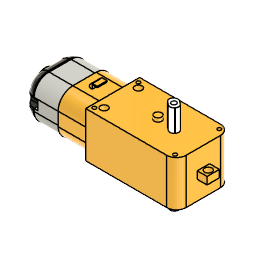
DC Motor (Autodesk Fusion 360 design; units mm, degrees)
part number: 2025-10-12-13-39-24-914
part number: 2025-10-12-13-42-40-722
part number: 2025-10-12-13-44-59-312
part number: 2025-10-12-15-17-17-342
part number: 2025-10-12-15-31-43-485
part number: 2025-10-12-15-34-23-255
part number: 2025-10-12-15-55-27-958
part number: 2025-10-12-16-01-49-874
Autodesk Fusion 360 part; units mm, degrees
sketch "Sketch1" plane through (0, 0, 0) normal (0, 1, 0) x (1, 0, 0)
  line L0 (18.5, 9.25) -> (-18.5, 9.25)
  line L1 (-18.5, 9.25) -> (-18.5, -9.25)
  line L2 (-18.5, -9.25) -> (18.5, -9.25)
  line L3 (18.5, -9.25) -> (18.5, 9.25)
  line L4 (18.5, 9.25) -> (-18.5, -9.25) construction
  line L5 (-18.5, 9.25) -> (18.5, -9.25) construction
  dimension "d1" = 37
  dimension "d2" = 18.5
  constraint horizontal L0
  constraint perpendicular L0 L1
  constraint parallel L0 L2
  constraint parallel L1 L3
  constraint coincident L4 origin
  constraint coincident L5 origin
  measures "d1" distance of L1.end L2.end
  measures "d2" distance of L0.start L2.end
extrude "Extrude1" add sketch "Sketch1" along normal blind 22 makes body 1
sketch "Sketch2" plane through (-18.5, 0, 0) normal (-1, 0, 0) x (0, -1, 0)
  line L0 (0, -9.25) -> (0, 9.25)
  line L1 (0, 9.25) -> (-22, 9.25)
  line L2 (-22, 9.25) -> (-22, -9.25)
  line L3 (-22, -9.25) -> (0, -9.25)
  line L4 (-0.25, -9.05) -> (-21.75, -9.05)
  line L5 (-21.75, -9.05) -> (-21.75, 8.45)
  line L6 (-21.75, 8.45) -> (-0.25, 8.45)
  line L7 (-0.25, 8.45) -> (-0.25, -9.05)
  line L8 (-0.25, -9.05) -> (-21.75, 8.45) construction
  line L9 (-21.75, -9.05) -> (-0.25, 8.45) construction
  point P0 (-11, -0.3)
  dimension "d5" = 21.5
  dimension "d6" = 17.5
  dimension "d7" = 0.25
  dimension "d8" = 0.2
  constraint horizontal L4
  constraint perpendicular L4 L5
  constraint parallel L4 L6
  constraint parallel L5 L7
  constraint coincident L8 P0
  constraint coincident L9 P0
  measures "d5" distance of L5.end L6.end
  measures "d6" distance of L4.start L6.end
  measures "d7" distance of L2 L5
  measures "d8" distance of L3 L4
extrude "Extrude1'" add sketch "Sketch2" along normal blind 11.5 separate body contours L4 L5 L6 L7 makes body 2 in component "Component"
sketch "Sketch3" plane through (-30, 0, 0) normal (-1, 0, 0) x (0, -1, 0)
  line L0 (-0.25, 8.45) -> (-21.75, 8.45)
  line L1 (-21.75, 8.45) -> (-21.75, -9.05)
  line L2 (-21.75, -9.05) -> (-0.25, -9.05)
  line L3 (-0.25, -9.05) -> (-0.25, 8.45)
  line L4 (-0.454, -8.785) -> (-21.454, -8.785)
  line L5 (-21.454, -8.785) -> (-21.454, 8.215)
  line L6 (-21.454, 8.215) -> (-0.454, 8.215)
  line L7 (-0.454, 8.215) -> (-0.454, -8.785)
  line L8 (-0.454, -8.785) -> (-21.454, 8.215) construction
  line L9 (-21.454, -8.785) -> (-0.454, 8.215) construction
  point P0 (-10.954, -0.285)
  dimension "d11" = 21
  dimension "d12" = 17
  dimension "d13" = 0.235
  dimension "d14" = 0.296
  constraint horizontal L4
  constraint perpendicular L4 L5
  constraint parallel L4 L6
  constraint parallel L5 L7
  constraint coincident L8 P0
  constraint coincident L9 P0
  measures "d11" distance of L5.end L6.end
  measures "d12" distance of L4.start L6.end
  measures "d13" distance of L0 L6
  measures "d14" distance of L1 L5
extrude "Extrude1''" add sketch "Sketch3" along normal blind 10 separate body contours L4 L5 L6 L7 makes body 3 in component "Component'"
fillet "Fillet1" radius 4 2 edges at (18.5, 0, 0) (18.5, 22, 0) on bodies 1
sketch "Sketch4" plane through (18.5, 0, 0) normal (1, 0, 0) x (0, 1, 0)
  line L0 (18, -9.25) -> (18, 9.25)
  line L1 (18, 9.25) -> (4, 9.25)
  line L2 (4, 9.25) -> (4, -9.25)
  line L3 (4, -9.25) -> (18, -9.25)
  line L4 (13.5, -1.5) -> (8.5, -1.5)
  line L5 (8.5, -1.5) -> (8.5, 1.5)
  line L6 (8.5, 1.5) -> (13.5, 1.5)
  line L7 (13.5, 1.5) -> (13.5, -1.5)
  line L8 (13.5, -1.5) -> (8.5, 1.5) construction
  line L9 (8.5, -1.5) -> (13.5, 1.5) construction
  point P0 (11, 0)
  dimension "d23" = 5
  dimension "d24" = 3
  constraint horizontal L4
  constraint perpendicular L4 L5
  constraint parallel L4 L6
  constraint parallel L5 L7
  constraint coincident L8 P0
  constraint coincident L9 P0
  measures "d23" distance of L5.end L6.end
  measures "d24" distance of L4.start L6.end
extrude "Extrude2" add sketch "Sketch4" along normal blind 4 contours L4 L5 L6 L7 bodies 1
sketch "Sketch5" plane through (0, 0, 1.5) normal (0, 0, 1) x (-1, 0, 0)
  line L0 (-18.5, -13.5) -> (-18.5, -8.5)
  line L1 (-18.5, -8.5) -> (-22.5, -8.5)
  line L2 (-22.5, -8.5) -> (-22.5, -13.5)
  line L3 (-22.5, -13.5) -> (-18.5, -13.5)
  circle A0 centre (-20.5, -11) radius 1.5
  dimension "d27" = 3
  measures "d27" diameter of A0
extrude "Extrude3" cut sketch "Sketch5" against normal blind 3 contours A0 bodies 1
sketch "Sketch7" plane through (0, 0, 9.25) normal (0, 0, 1) x (-1, 0, 0)
  arc A0 (-18.5, -18) -> (-14.5, -22) centre (-14.5, -18) ccw
  line L0 (-14.5, -22) -> (18.5, -22)
  line L1 (18.5, -22) -> (18.5, 0)
  line L2 (18.5, 0) -> (-14.5, 0)
  arc A1 (-14.5, 0) -> (-18.5, -4) centre (-14.5, -4) ccw
  line L3 (-18.5, -4) -> (-18.5, -18)
  line L4 (-7.3842, -8.0793) -> (-3.453, -11.169)
  line L5 (-3.453, -11.169) -> (-5.6158, -13.9207)
  line L6 (-5.6158, -13.9207) -> (-9.547, -10.831)
  line L7 (-9.547, -10.831) -> (-7.3842, -8.0793)
  line L8 (-7.3842, -8.0793) -> (-5.6158, -13.9207) construction
  line L9 (-3.453, -11.169) -> (-9.547, -10.831) construction
  point P0 (-6.5, -11)
  dimension "d32" = 5
  dimension "d33" = 3.5
  dimension "d34" = 12
  dimension "d35" = 11
  constraint perpendicular L4 L5
  constraint parallel L4 L6
  constraint parallel L5 L7
  constraint coincident L8 P0
  constraint coincident L9 P0
  measures "d32" distance of L5.end L6.end
  measures "d33" distance of L4.start L6.end
  measures "d34" distance of L3 P0
  measures "d35" distance of L2 P0
extrude "Extrude4" add sketch "Sketch7" along normal blind 9 separate body contours L4 L5 L6 L7 makes body 4
extrude "Extrude5" add 1 faces at (5.4843, 11.0563, 18.25) along direction (0, 0, -1) blind 36.5 on bodies 4 bodies 1 4
fillet "Fillet2" radius 1.65 8 edges at (7.3842, 8.0793, 13.75) (9.547, 10.831, 13.75) (3.453, 11.169, 13.75) (5.6158, 13.9207, 13.75) (9.547, 10.831, -13.75) (5.6158, 13.9207, -13.75) (3.453, 11.169, -13.75) (7.3842, 8.0793, -13.75) on bodies 1
sketch "Sketch8" plane through (0, 0, 9.25) normal (0, 0, 1) x (-1, 0, 0)
  line L0 (-8.5274, -9.5338) -> (-8.4038, -9.3765)
  arc A0 (-6.0869, -9.0989) -> (-8.4038, -9.3765) centre (-7.1065, -10.3961) ccw
  line L1 (-6.0869, -9.0989) -> (-4.7503, -10.1494)
  arc A1 (-4.4726, -12.4662) -> (-4.7503, -10.1494) centre (-5.7699, -11.4466) ccw
  line L2 (-4.4726, -12.4662) -> (-4.5962, -12.6235)
  arc A2 (-6.9131, -12.9011) -> (-4.5962, -12.6235) centre (-5.8935, -11.6039) ccw
  line L3 (-6.9131, -12.9011) -> (-8.2497, -11.8506)
  arc A3 (-8.5274, -9.5338) -> (-8.2497, -11.8506) centre (-7.2301, -10.5534) ccw
  arc A4 (-18.5, -18) -> (-14.5, -22) centre (-14.5, -18) ccw
  line L4 (-14.5, -22) -> (18.5, -22)
  line L5 (18.5, -22) -> (18.5, 0)
  line L6 (18.5, 0) -> (-14.5, 0)
  arc A5 (-14.5, 0) -> (-18.5, -4) centre (-14.5, -4) ccw
  line L7 (-18.5, -4) -> (-18.5, -18)
  circle A6 centre (17, -20) radius 0.75
  circle A7 centre (-16, -20) radius 0.75
  circle A8 centre (-16, -2) radius 0.75
  circle A9 centre (17, -2) radius 0.75
  dimension "d42" = 1.5
  dimension "d43" = 1.5
  dimension "d44" = 1.5
  dimension "d45" = 1.5
  measures "d42" diameter of A6
  measures "d43" diameter of A7
  measures "d44" diameter of A8
  measures "d45" diameter of A9
extrude "Extrude6" cut sketch "Sketch8" against normal blind 5 contours A6 | A7 | A8 | A9 bodies 1
sketch "Sketch9" plane through (0, 0, 9.25) normal (0, 0, 1) x (-1, 0, 0)
  circle A0 centre (-16, -20) radius 0.75
  circle A1 centre (-16, -2) radius 0.75
  circle A2 centre (17, -20) radius 0.75
  circle A3 centre (17, -2) radius 0.75
  line L0 (-8.5274, -9.5338) -> (-8.4038, -9.3765)
  arc A4 (-6.0869, -9.0989) -> (-8.4038, -9.3765) centre (-7.1065, -10.3961) ccw
  line L1 (-6.0869, -9.0989) -> (-4.7503, -10.1494)
  arc A5 (-4.4726, -12.4662) -> (-4.7503, -10.1494) centre (-5.7699, -11.4466) ccw
  line L2 (-4.4726, -12.4662) -> (-4.5962, -12.6235)
  arc A6 (-6.9131, -12.9011) -> (-4.5962, -12.6235) centre (-5.8935, -11.6039) ccw
  line L3 (-6.9131, -12.9011) -> (-8.2497, -11.8506)
  arc A7 (-8.5274, -9.5338) -> (-8.2497, -11.8506) centre (-7.2301, -10.5534) ccw
  arc A8 (-18.5, -18) -> (-14.5, -22) centre (-14.5, -18) ccw
  line L4 (-14.5, -22) -> (18.5, -22)
  line L5 (18.5, -22) -> (18.5, 0)
  line L6 (18.5, 0) -> (-14.5, 0)
  arc A9 (-14.5, 0) -> (-18.5, -4) centre (-14.5, -4) ccw
  line L7 (-18.5, -4) -> (-18.5, -18)
  circle A10 centre (15, -18) radius 1.5
  circle A11 centre (-14, -18) radius 1.5
  circle A12 centre (-14, -4) radius 1.5
  circle A13 centre (15, -4) radius 1.5
  dimension "d48" = 3
  dimension "d49" = 3
  dimension "d50" = 3
  dimension "d51" = 3
  measures "d48" diameter of A10
  measures "d49" diameter of A11
  measures "d50" diameter of A12
  measures "d51" diameter of A13
extrude "Extrude7" cut sketch "Sketch9" against normal blind 5 contours A10 | A13 bodies 1
extrude "Extrude8" cut 2 faces at (-15.3832, 18.562, 4.25) (-15.237, 3.6091, 4.25) along direction (0, 0, -1) blind 10 on bodies 1 bodies 1
extrude "Extrude9" cut 2 faces at (-15.3832, 18.562, -5.75) (-15.237, 3.6091, -5.75) along direction (0, 0, -1) blind 25 on bodies 1 bodies 1
sketch "Sketch10" plane through (0, 0, -9.25) normal (0, 0, -1) x (1, 0, 0)
  circle A0 centre (-15, -18) radius 1.5
  circle A1 centre (-15, -4) radius 1.5
  line L0 (4.5962, -12.6235) -> (4.4726, -12.4662)
  arc A2 (4.7503, -10.1494) -> (4.4726, -12.4662) centre (5.7699, -11.4466) ccw
  line L1 (4.7503, -10.1494) -> (6.0869, -9.0989)
  arc A3 (8.4038, -9.3765) -> (6.0869, -9.0989) centre (7.1065, -10.3961) ccw
  line L2 (8.4038, -9.3765) -> (8.5274, -9.5338)
  arc A4 (8.2497, -11.8506) -> (8.5274, -9.5338) centre (7.2301, -10.5534) ccw
  line L3 (8.2497, -11.8506) -> (6.9131, -12.9011)
  arc A5 (4.5962, -12.6235) -> (6.9131, -12.9011) centre (5.8935, -11.6039) ccw
  arc A6 (14.5, -22) -> (18.5, -18) centre (14.5, -18) ccw
  line L4 (18.5, -18) -> (18.5, -4)
  arc A7 (18.5, -4) -> (14.5, 0) centre (14.5, -4) ccw
  line L5 (14.5, 0) -> (-18.5, 0)
  line L6 (-18.5, 0) -> (-18.5, -22)
  line L7 (-18.5, -22) -> (14.5, -22)
  circle A8 centre (-16.4, -6.9) radius 2
  circle A9 centre (-16.4, -15.1) radius 2
  dimension "d58" = 4
  dimension "d59" = 4
  measures "d58" diameter of A8
  measures "d59" diameter of A9
extrude "Extrude10" cut sketch "Sketch10" against normal blind 3 contours A0 A9 | A1 A8 picked at (-16.6375, -14.3779) picked at (-16.6375, -7.6221) bodies 1
sketch "Sketch11" plane through (-40, 0, 0) normal (-1, 0, 0) x (0, -1, 0)
  line L0 (-0.454, 8.215) -> (-21.454, 8.215)
  line L1 (-21.454, 8.215) -> (-21.454, -8.785)
  line L2 (-21.454, -8.785) -> (-0.454, -8.785)
  line L3 (-0.454, -8.785) -> (-0.454, 8.215)
  line L4 (-0.654, -8.685) -> (-21.254, -8.685)
  line L5 (-21.254, -8.685) -> (-21.254, 8.115)
  line L6 (-21.254, 8.115) -> (-0.654, 8.115)
  line L7 (-0.654, 8.115) -> (-0.654, -8.685)
  line L8 (-0.654, -8.685) -> (-21.254, 8.115) construction
  line L9 (-21.254, -8.685) -> (-0.654, 8.115) construction
  point P0 (-10.954, -0.285)
  dimension "d62" = 0.1
  dimension "d63" = 0.2
  dimension "d64" = 0.2
  dimension "d65" = 0.1
  constraint horizontal L4
  constraint perpendicular L4 L5
  constraint parallel L4 L6
  constraint parallel L5 L7
  constraint coincident L8 P0
  constraint coincident L9 P0
  measures "d62" distance of L0 L6
  measures "d63" distance of L3 L7
  measures "d64" distance of L1 L5
  measures "d65" distance of L2 L4
extrude "Extrude1'''" add sketch "Sketch11" along normal blind 4 separate body contours L4 L5 L6 L7 makes body 5 in component "Component''"
sketch "Sketch12" plane through (0, 21.454, 0) normal (0, 1, 0) x (-1, 0, 0)
  line L0 (30, 8.215) -> (30, -8.785)
  line L1 (30, -8.785) -> (40, -8.785)
  line L2 (40, -8.785) -> (40, 8.215)
  line L3 (40, 8.215) -> (30, 8.215)
  line L4 (45.5, -1.75) -> (38.5, -1.75)
  line L5 (38.5, -1.75) -> (38.5, 1.75)
  line L6 (38.5, 1.75) -> (45.5, 1.75)
  line L7 (45.5, 1.75) -> (45.5, -1.75)
  line L8 (45.5, -1.75) -> (38.5, 1.75) construction
  line L9 (38.5, -1.75) -> (45.5, 1.75) construction
  point P0 (42, 0)
  dimension "d68" = 7
  dimension "d69" = 3.5
  constraint horizontal L4
  constraint perpendicular L4 L5
  constraint parallel L4 L6
  constraint parallel L5 L7
  constraint coincident L8 P0
  constraint coincident L9 P0
  measures "d68" distance of L5.end L6.end
  measures "d69" distance of L4.start L6.end
extrude "Extrude2'" cut sketch "Sketch12" against normal blind 2.5 contours L2 L4 L6 L7 | L2 L4 L5 L6 bodies 3 in component "Component'"
extrude "Extrude2''" cut sketch "Sketch12" against normal blind 2.5 contours L2 L4 L6 L7 | L2 L4 L5 L6 bodies 5 in component "Component''"
sketch "Sketch13" plane through (0, 0.454, 0) normal (0, -1, 0) x (1, 0, 0)
  line L0 (-30, -8.785) -> (-30, 8.215)
  line L1 (-30, 8.215) -> (-40, 8.215)
  line L2 (-40, 8.215) -> (-40, -8.785)
  line L3 (-40, -8.785) -> (-30, -8.785)
  line L4 (-38.4787, -1.7463) -> (-45.4787, -1.7463)
  line L5 (-45.4787, -1.7463) -> (-45.4787, 1.7537)
  line L6 (-45.4787, 1.7537) -> (-38.4787, 1.7537)
  line L7 (-38.4787, 1.7537) -> (-38.4787, -1.7463)
  line L8 (-38.4787, -1.7463) -> (-45.4787, 1.7537) construction
  line L9 (-45.4787, -1.7463) -> (-38.4787, 1.7537) construction
  point P0 (-41.9787, 0.0037)
  dimension "d74" = 7
  dimension "d75" = 3.5
  constraint horizontal L4
  constraint perpendicular L4 L5
  constraint parallel L4 L6
  constraint parallel L5 L7
  constraint coincident L8 P0
  constraint coincident L9 P0
  measures "d74" distance of L5.end L6.end
  measures "d75" distance of L4.start L6.end
extrude "Extrude3'" cut sketch "Sketch13" against normal blind 2.5 contours L2 L4 L5 L6 | L2 L4 L6 L7 bodies 3 in component "Component'"
extrude "Extrude3''" cut sketch "Sketch13" against normal blind 2.5 contours L2 L4 L5 L6 | L2 L4 L6 L7 bodies 5 in component "Component''"
fillet "Fillet2'" radius 6 4 edges at (-35, 0.454, 8.215) (-35, 21.454, 8.215) (-35, 21.454, -8.785) (-35, 0.454, -8.785) on bodies 3 in component "Component'"
fillet "Fillet1'" radius 6 4 edges at (-42, 0.654, 8.115) (-42, 0.654, -8.685) (-42, 21.254, 8.115) (-42, 21.254, -8.685) on bodies 5 in component "Component''"
fillet "Fillet2''" radius 6 4 edges at (-24.25, 0.25, 8.45) (-24.25, 0.25, -9.05) (-24.25, 21.75, 8.45) (-24.25, 21.75, -9.05) on bodies 2 in component "Component"
sketch "Sketch14" plane through (-44, 0, 0) normal (-1, 0, 0) x (0, -1, 0)
  arc A0 (-21.254, -2.685) -> (-15.254, -8.685) centre (-15.254, -2.685) ccw
  line L0 (-15.254, -8.685) -> (-6.654, -8.685)
  arc A1 (-6.654, -8.685) -> (-0.654, -2.685) centre (-6.654, -2.685) ccw
  line L1 (-0.654, -2.685) -> (-0.654, -1.7463)
  line L2 (-0.654, -1.7463) -> (-2.954, -1.7463)
  line L3 (-2.954, -1.7463) -> (-2.954, 1.7537)
  line L4 (-2.954, 1.7537) -> (-0.654, 1.7537)
  line L5 (-0.654, 1.7537) -> (-0.654, 2.115)
  arc A2 (-0.654, 2.115) -> (-6.654, 8.115) centre (-6.654, 2.115) ccw
  line L6 (-6.654, 8.115) -> (-15.254, 8.115)
  arc A3 (-15.254, 8.115) -> (-21.254, 2.115) centre (-15.254, 2.115) ccw
  line L7 (-21.254, 2.115) -> (-21.254, 1.75)
  line L8 (-21.254, 1.75) -> (-18.954, 1.75)
  line L9 (-18.954, 1.75) -> (-18.954, -1.75)
  line L10 (-18.954, -1.75) -> (-21.254, -1.75)
  line L11 (-21.254, -1.75) -> (-21.254, -2.685)
  circle A4 centre (-11, 0) radius 4.5
  dimension "d86" = 9
  measures "d86" diameter of A4
extrude "Extrude1''''" add sketch "Sketch14" along normal blind 2 separate body contours A4 makes body 6 in component "Component'''"
sketch "Sketch15" plane through (-46, 0, 0) normal (-1, 0, 0) x (0, -1, 0)
  circle A0 centre (-11, 0) radius 4.5
  circle A1 centre (-11, 0) radius 1.5
  dimension "d89" = 3
  constraint concentric A0 A1
  measures "d89" diameter of A1
extrude "Extrude2'''" cut sketch "Sketch15" against normal blind 1 contours A1 bodies 6 in component "Component'''"
sketch "Sketch16" plane through (-45, 0, 0) normal (-1, 0, 0) x (0, -1, 0)
  circle A0 centre (-11, 0) radius 1.5
  circle A1 centre (-11, 0) radius 0.5
  dimension "d92" = 1
  constraint concentric A0 A1
  measures "d92" diameter of A1
extrude "Extrude1'''''" add sketch "Sketch16" along normal blind 2 separate body contours A1 makes body 7 in component "Component''''"
sketch "Sketch17" plane through (-46, 0, 0) normal (-1, 0, 0) x (0, -1, 0)
  circle A0 centre (-11, 0) radius 1.5
  circle A1 centre (-11, 0) radius 4.5
  line L0 (-8.2595, 2.0042) -> (-13.7595, 2.0042)
  line L1 (-13.7595, 2.0042) -> (-13.7595, 3.0042)
  line L2 (-13.7595, 3.0042) -> (-8.2595, 3.0042)
  line L3 (-8.2595, 3.0042) -> (-8.2595, 2.0042)
  line L4 (-8.2595, 2.0042) -> (-13.7595, 3.0042) construction
  line L5 (-13.7595, 2.0042) -> (-8.2595, 3.0042) construction
  point P0 (-11.0095, 2.5042)
  dimension "d95" = 5.5
  dimension "d96" = 1
  constraint horizontal L0
  constraint perpendicular L0 L1
  constraint parallel L0 L2
  constraint parallel L1 L3
  constraint coincident L4 P0
  constraint coincident L5 P0
  measures "d95" distance of L1.end L2.end
  measures "d96" distance of L0.end L1.end
extrude "Extrude4'" cut sketch "Sketch17" against normal blind 3 contours L0 L1 L2 L3 bodies 5 in component "Component''"
extrude "Extrude3'''" cut sketch "Sketch17" against normal blind 3 contours L0 L1 L2 L3 bodies 6 in component "Component'''"
sketch "Sketch18" plane through (-46, 0, 0) normal (-1, 0, 0) x (0, -1, 0)
  line L0 (-13.7595, 2.0042) -> (-13.7595, 3.0042)
  line L1 (-13.7595, 3.0042) -> (-8.2595, 3.0042)
  line L2 (-8.2595, 3.0042) -> (-8.2595, 2.0042)
  line L3 (-8.2595, 2.0042) -> (-13.7595, 2.0042)
  circle A0 centre (-11, 0) radius 1.5
  circle A1 centre (-11, 0) radius 4.5
  line L4 (-14.0414, -3.3166) -> (-7.9586, -3.3166)
  constraint coincident A1 L4.start
  constraint coincident A1 L4.end
  constraint horizontal L4
extrude "Extrude4''" cut sketch "Sketch18" against normal blind 2 contours A1 L4 picked at (-11.8392, -3.4544) bodies 6 in component "Component'''"
fillet "Fillet2'''" radius 3.5 10 edges at (-44, 21.254, 1.9325) (-44, 19.4966, 6.3576) (-44, 10.954, 8.115) (-44, 2.4114, 6.3576) (-44, 0.654, 1.9344) (-44, 0.654, -2.2156) (-44, 2.4114, -6.9276) (-44, 10.954, -8.685) (-44, 19.4966, -6.9276) (-44, 21.254, -2.2175) on bodies 5 in component "Component''"
sketch "Sketch19" plane through (0, 0, 8.45) normal (0, 0, 1) x (-1, 0, 0)
  line L0 (18.5, -15.75) -> (30, -15.75)
  line L1 (30, -15.75) -> (30, -6.25)
  line L2 (30, -6.25) -> (18.5, -6.25)
  line L3 (18.5, -6.25) -> (18.5, -15.75)
  line L4 (26, -13.0103) -> (24.8, -13.0103)
  line L5 (24.8, -13.0103) -> (24.8, -9.0103)
  line L6 (24.8, -9.0103) -> (26, -9.0103)
  line L7 (26, -9.0103) -> (26, -13.0103)
  line L8 (26, -13.0103) -> (24.8, -9.0103) construction
  line L9 (24.8, -13.0103) -> (26, -9.0103) construction
  point P0 (25.4, -11.0103)
  dimension "d105" = 4
  dimension "d106" = 4
  dimension "d107" = 1.2
  constraint horizontal L4
  constraint perpendicular L4 L5
  constraint parallel L4 L6
  constraint parallel L5 L7
  constraint coincident L8 P0
  constraint coincident L9 P0
  measures "d105" distance of L4.end L5.end
  measures "d106" distance of L1 L7
  measures "d107" distance of L5.end L6.end
extrude "Extrude2''''" add sketch "Sketch19" along normal blind 2 contours L4 L5 L6 L7 bodies 2 in component "Component"
sketch "Sketch20" plane through (-24.8, 0, 0) normal (1, 0, 0) x (0, 1, 0)
  line L0 (9.0103, 8.45) -> (13.0103, 8.45)
  line L1 (13.0103, 8.45) -> (13.0103, 10.45)
  line L2 (13.0103, 10.45) -> (9.0103, 10.45)
  line L3 (9.0103, 10.45) -> (9.0103, 8.45)
  line L4 (13.0147, 9.949) -> (9.0147, 9.949)
  line L5 (9.0147, 9.949) -> (9.0147, 10.449)
  line L6 (9.0147, 10.449) -> (13.0147, 10.449)
  line L7 (13.0147, 10.449) -> (13.0147, 9.949)
  line L8 (13.0147, 9.949) -> (9.0147, 10.449) construction
  line L9 (9.0147, 9.949) -> (13.0147, 10.449) construction
  point P0 (11.0147, 10.199)
  dimension "d110" = 4
  dimension "d111" = 0.5
  dimension "d112" = 0.001
  constraint horizontal L4
  constraint perpendicular L4 L5
  constraint parallel L4 L6
  constraint parallel L5 L7
  constraint coincident L8 P0
  constraint coincident L9 P0
  measures "d110" distance of L5.end L6.end
  measures "d111" distance of L4.end L5.end
  measures "d112" distance of L2 L6
extrude "Extrude3''''" add sketch "Sketch20" along normal blind 2 contours L1 L4 L5 L6 bodies 2 in component "Component"
chamfer "Chamfer1" distance 1 angle 45 1 edges at (-26, 11.0103, 10.45) on bodies 2 in component "Component"
sketch "Sketch21" plane through (0, 0, -9.05) normal (0, 0, -1) x (1, 0, 0)
  line L0 (-30, -15.75) -> (-18.5, -15.75)
  line L1 (-18.5, -15.75) -> (-18.5, -6.25)
  line L2 (-18.5, -6.25) -> (-30, -6.25)
  line L3 (-30, -6.25) -> (-30, -15.75)
  line L4 (-26, -9.0505) -> (-24.8, -9.0505)
  line L5 (-24.8, -9.0505) -> (-24.8, -13.0505)
  line L6 (-24.8, -13.0505) -> (-26, -13.0505)
  line L7 (-26, -13.0505) -> (-26, -9.0505)
  line L8 (-26, -9.0505) -> (-24.8, -13.0505) construction
  line L9 (-24.8, -9.0505) -> (-26, -13.0505) construction
  point P0 (-25.4, -11.0505)
  dimension "d116" = 4
  dimension "d117" = 1.2
  dimension "d118" = 4
  constraint horizontal L4
  constraint perpendicular L4 L5
  constraint parallel L4 L6
  constraint parallel L5 L7
  constraint coincident L8 P0
  constraint coincident L9 P0
  measures "d116" distance of L4.start L6.end
  measures "d117" distance of L4.start L4.end
  measures "d118" distance of L3 L7
extrude "Extrude4'''" add sketch "Sketch21" along normal blind 2 contours L4 L5 L6 L7 bodies 2 in component "Component"
sketch "Sketch22" plane through (-24.8, 0, 0) normal (1, 0, 0) x (0, 1, 0)
  line L0 (13.0505, -9.05) -> (9.0505, -9.05)
  line L1 (9.0505, -9.05) -> (9.0505, -11.05)
  line L2 (9.0505, -11.05) -> (13.0505, -11.05)
  line L3 (13.0505, -11.05) -> (13.0505, -9.05)
  line L4 (9.0605, -10.544) -> (13.0605, -10.544)
  line L5 (13.0605, -10.544) -> (13.0605, -11.044)
  line L6 (13.0605, -11.044) -> (9.0605, -11.044)
  line L7 (9.0605, -11.044) -> (9.0605, -10.544)
  line L8 (9.0605, -10.544) -> (13.0605, -11.044) construction
  line L9 (13.0605, -10.544) -> (9.0605, -11.044) construction
  point P0 (11.0605, -10.794)
  dimension "d121" = 4
  dimension "d122" = 0.5
  constraint horizontal L4
  constraint perpendicular L4 L5
  constraint parallel L4 L6
  constraint parallel L5 L7
  constraint coincident L8 P0
  constraint coincident L9 P0
  measures "d121" distance of L5.end L6.end
  measures "d122" distance of L4.start L6.end
extrude "Extrude5'" add sketch "Sketch22" along normal blind 2 contours L3 L4 L6 L7 bodies 2 in component "Component"
chamfer "Chamfer2" distance 1 angle 45 1 edges at (-26, 11.0505, -11.05) on bodies 2 in component "Component"
sketch "Sketch23" plane through (0, 0, -6.25) normal (0, 0, -1) x (1, 0, 0)
  arc A0 (-16.1918, -4.9109) -> (-14.972, -5.4997) centre (-16.4, -6.9) ccw
  arc A1 (-16.1918, -4.9109) -> (-14.972, -5.4997) centre (-15, -4) ccw
  circle A2 centre (-16.4, -6.9) radius 1.5
  dimension "d126" = 3
  constraint concentric A0 A2
  measures "d126" diameter of A2
extrude "Extrude1''''''" add sketch "Sketch23" along normal blind 1.5 separate body contours A2 makes body 8 in component "Component'''''"
sketch "Sketch24" plane through (0, 0, -7.75) normal (0, 0, -1) x (1, 0, 0)
  circle A0 centre (-16.4, -6.9) radius 1.5
  line L0 (-16.15, -8.15) -> (-16.65, -8.15)
  line L1 (-16.65, -8.15) -> (-16.65, -5.65)
  line L2 (-16.65, -5.65) -> (-16.15, -5.65)
  line L3 (-16.15, -5.65) -> (-16.15, -8.15)
  line L4 (-16.15, -8.15) -> (-16.65, -5.65) construction
  line L5 (-16.65, -8.15) -> (-16.15, -5.65) construction
  line L6 (-15.15, -7.15) -> (-17.65, -7.15)
  line L7 (-17.65, -7.15) -> (-17.65, -6.65)
  line L8 (-17.65, -6.65) -> (-15.15, -6.65)
  line L9 (-15.15, -6.65) -> (-15.15, -7.15)
  line L10 (-15.15, -7.15) -> (-17.65, -6.65) construction
  line L11 (-17.65, -7.15) -> (-15.15, -6.65) construction
  point P0 (-16.4, -6.9)
  point P1 (-16.4, -6.9)
  dimension "d129" = 2.5
  dimension "d130" = 0.5
  dimension "d131" = 2.5
  dimension "d132" = 0.5
  constraint horizontal L0
  constraint perpendicular L0 L1
  constraint parallel L0 L2
  constraint parallel L1 L3
  constraint coincident L4 P1
  constraint coincident L5 P1
  constraint coincident P0 A0.centre
  constraint horizontal L6
  constraint perpendicular L6 L7
  constraint parallel L6 L8
  constraint parallel L7 L9
  constraint coincident L10 P1
  constraint coincident L11 P1
  constraint coincident P1 P0
  measures "d129" distance of L0.start L2.end
  measures "d130" distance of L0.start L0.end
  measures "d131" distance of L7.end L8.end
  measures "d132" distance of L6.start L8.end
extrude "Extrude2'''''" add sketch "Sketch24" along normal blind 0.3 bodies 8 in component "Component'''''"
copy_body "CopyPasteBodies1" bodies 8 makes body 9
move_body "Move1" bodies 9 to x (1, 0, 0) y (0, 1, 0) z (0, 0, 1) at (0, 8.25, 0)
sketch "Sketch25" plane through (0, 0, 9.25) normal (0, 0, 1) x (-1, 0, 0)
  circle A0 centre (15, -18) radius 1.5
  circle A1 centre (15, -4) radius 1.5
  circle A2 centre (-16, -20) radius 0.75
  circle A3 centre (-16, -2) radius 0.75
  circle A4 centre (17, -20) radius 0.75
  circle A5 centre (17, -2) radius 0.75
  line L0 (-8.5274, -9.5338) -> (-8.4038, -9.3765)
  arc A6 (-6.0869, -9.0989) -> (-8.4038, -9.3765) centre (-7.1065, -10.3961) ccw
  line L1 (-6.0869, -9.0989) -> (-4.7503, -10.1494)
  arc A7 (-4.4726, -12.4662) -> (-4.7503, -10.1494) centre (-5.7699, -11.4466) ccw
  line L2 (-4.4726, -12.4662) -> (-4.5962, -12.6235)
  arc A8 (-6.9131, -12.9011) -> (-4.5962, -12.6235) centre (-5.8935, -11.6039) ccw
  line L3 (-6.9131, -12.9011) -> (-8.2497, -11.8506)
  arc A9 (-8.5274, -9.5338) -> (-8.2497, -11.8506) centre (-7.2301, -10.5534) ccw
  arc A10 (-18.5, -18) -> (-14.5, -22) centre (-14.5, -18) ccw
  line L4 (-14.5, -22) -> (18.5, -22)
  line L5 (18.5, -22) -> (18.5, 0)
  line L6 (18.5, 0) -> (-14.5, 0)
  arc A11 (-14.5, 0) -> (-18.5, -4) centre (-14.5, -4) ccw
  line L7 (-18.5, -4) -> (-18.5, -18)
  circle A12 centre (0, -11) radius 1.5
  dimension "d135" = 3
  measures "d135" diameter of A12
extrude "Extrude11" add sketch "Sketch25" along normal blind 1.5 contours A12 bodies 1
sketch "Sketch26" plane through (0, 0, -8.785) normal (0, 0, -1) x (1, 0, 0)
  line L0 (-30, -6.454) -> (-40, -6.454)
  line L1 (-40, -6.454) -> (-40, -15.454)
  line L2 (-40, -15.454) -> (-30, -15.454)
  line L3 (-30, -15.454) -> (-30, -6.454)
  line L4 (-41, -7.454) -> (-39, -7.454)
  line L5 (-39, -7.454) -> (-39, -14.454)
  line L6 (-39, -14.454) -> (-41, -14.454)
  line L7 (-41, -14.454) -> (-41, -7.454)
  line L8 (-41, -7.454) -> (-39, -14.454) construction
  line L9 (-39, -7.454) -> (-41, -14.454) construction
  point P0 (-40, -10.954)
  dimension "d138" = 7
  dimension "d139" = 2
  constraint horizontal L4
  constraint perpendicular L4 L5
  constraint parallel L4 L6
  constraint parallel L5 L7
  constraint coincident L8 P0
  constraint coincident L9 P0
  measures "d138" distance of L4.start L6.end
  measures "d139" distance of L5.end L6.end
extrude "Extrude1'''''''" add sketch "Sketch26" along normal blind 0.5 separate body contours L1 L4 L5 L6 | L1 L4 L6 L7 makes body 10 in component "Component''''''"
sketch "Sketch27" plane through (0, 0, -9.285) normal (0, 0, -1) x (1, 0, 0)
  line L0 (-41, -14.454) -> (-39, -14.454)
  line L1 (-39, -14.454) -> (-39, -7.454)
  line L2 (-39, -7.454) -> (-41, -7.454)
  line L3 (-41, -7.454) -> (-41, -14.454)
  circle A0 centre (-40, -13.5) radius 0.75
  circle A1 centre (-40, -8.5) radius 0.75
  dimension "d142" = 1.5
  dimension "d143" = 1.5
  measures "d142" diameter of A0
  measures "d143" diameter of A1
extrude "Extrude3'''''" add sketch "Sketch27" along normal blind 0.75 contours A0 | A1 bodies 10 in component "Component''''''"
fillet "Fillet2''''" radius 0.7 2 edges at (-40.6992, 8.7712, -10.035) (-40.6992, 13.7712, -10.035) on bodies 10 in component "Component''''''"
sketch "Sketch28" plane through (0, 0, -18.25) normal (0, 0, -1) x (1, 0, 0)
  arc A0 (8.4038, -9.3765) -> (6.0869, -9.0989) centre (7.1065, -10.3961) ccw
  line L0 (6.0869, -9.0989) -> (4.7503, -10.1494)
  arc A1 (4.7503, -10.1494) -> (4.4726, -12.4662) centre (5.7699, -11.4466) ccw
  line L1 (4.4726, -12.4662) -> (4.5962, -12.6235)
  arc A2 (4.5962, -12.6235) -> (6.9131, -12.9011) centre (5.8935, -11.6039) ccw
  line L2 (6.9131, -12.9011) -> (8.2497, -11.8506)
  arc A3 (8.2497, -11.8506) -> (8.5274, -9.5338) centre (7.2301, -10.5534) ccw
  line L3 (8.5274, -9.5338) -> (8.4038, -9.3765)
  circle A4 centre (6.5, -11) radius 1
  dimension "d152" = 2
  measures "d152" diameter of A4
extrude "Extrude12" cut sketch "Sketch28" against normal blind 10 contours A4 bodies 1
sketch "Sketch29" plane through (0, 0, 18.25) normal (0, 0, 1) x (-1, 0, 0)
  arc A0 (-6.9131, -12.9011) -> (-4.5962, -12.6235) centre (-5.8935, -11.6039) ccw
  line L0 (-4.5962, -12.6235) -> (-4.4726, -12.4662)
  arc A1 (-4.4726, -12.4662) -> (-4.7503, -10.1494) centre (-5.7699, -11.4466) ccw
  line L1 (-4.7503, -10.1494) -> (-6.0869, -9.0989)
  arc A2 (-6.0869, -9.0989) -> (-8.4038, -9.3765) centre (-7.1065, -10.3961) ccw
  line L2 (-8.4038, -9.3765) -> (-8.5274, -9.5338)
  arc A3 (-8.5274, -9.5338) -> (-8.2497, -11.8506) centre (-7.2301, -10.5534) ccw
  line L3 (-8.2497, -11.8506) -> (-6.9131, -12.9011)
  circle A4 centre (-6.5, -11) radius 1
  dimension "d155" = 2
  measures "d155" diameter of A4
extrude "Extrude13" cut sketch "Sketch29" against normal blind 10 contours A4 bodies 1
component "Component" placed x (1, 0, 0) y (0, 1, 0) z (0, 0, 1) at (0, 0, 0)
component "Component'" placed x (1, 0, 0) y (0, 1, 0) z (0, 0, 1) at (0, 0, 0)
component "Component''" placed x (1, 0, 0) y (0, 1, 0) z (0, 0, 1) at (0, 0, 0)
component "Component'''" placed x (1, 0, 0) y (0, 1, 0) z (0, 0, 1) at (0, 0, 0)
component "Component''''" placed x (1, 0, 0) y (0, 1, 0) z (0, 0, 1) at (0, 0, 0)
component "Component'''''" placed x (1, 0, 0) y (0, 1, 0) z (0, 0, 1) at (0, 0, 0)
component "Component''''''" placed x (1, 0, 0) y (0, 1, 0) z (0, 0, 1) at (0, 0, 0)
